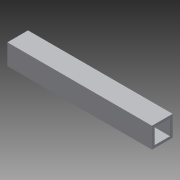
# Autodesk Inventor part: Box 7 inch
Saved by Autodesk Inventor 2014 (Build 180170000, 170)
## iProperties
Created: 2014-02-25
Part Number: Box 7 inch
Material: Aluminum 6061
Document SubType Name: Modeling
Designer: Nitesh
Density: 2.71 g/cm^3
Appearance: Aluminum - Flat
Mass: 136.002 g
Surface Area: 321.774 cm^2
Volume: 50.1854 cm^3
Author: Nitesh
Autodesk Inventor part; units mm, degrees
ref_plane "YZ Plane" through (0, 0, 0) normal (1, 0, 0) x (0, 1, 0)
ref_plane "XZ Plane" through (0, 0, 0) normal (0, 1, 0) x (-1, 0, 0)
ref_plane "XY Plane" through (0, 0, 0) normal (0, 0, 1) x (1, 0, 0)
sketch "Sketch1" plane through (0, 0, 0) normal (1, 0, 0) x (0, 1, 0)
  line L0 (0, 0) -> (25.4, 0)
  line L1 (25.4, 0) -> (25.4, 25.4)
  line L2 (25.4, 25.4) -> (0, 25.4)
  line L3 (0, 25.4) -> (0, 0)
  line L4 (3.175, 22.225) -> (22.225, 22.225)
  line L5 (22.225, 22.225) -> (22.225, 3.175)
  line L6 (22.225, 3.175) -> (3.175, 3.175)
  line L7 (3.175, 3.175) -> (3.175, 22.225)
  dimension "d0" = 25.4
  dimension "d1" = 25.4
  dimension "d2" = 3.175
  constraints: 16 end point, 4 parallel, 2 perpendicular, 1 horizontal, 3 other
  measures "d0" distance of L2.end L0.start
  measures "d1" distance of L1.end L2.end
  measures "d2" distance between parallel lines of L2 L4
extrude "Extrusion1" add sketch "Sketch1" along normal blind 177.8
body "Solid1"
